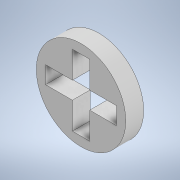
# Autodesk Inventor part: rod_7
Saved by Autodesk Inventor 2022 (Build 260153000, 153)
## iProperties
Created: 2023-04-14
Part Number: rod_7
Material: 一般
Document SubType Name: Modeling
Designer: Johnny Jou
Density: 1 g/cm^3
Appearance: 預設
Author: Johnny Jou
Autodesk Inventor part; units mm, degrees
ref_plane "YZ Plane" through (0, 0, 0) normal (1, 0, 0) x (0, 1, 0)
ref_plane "XZ Plane" through (0, 0, 0) normal (0, 1, 0) x (-1, 0, 0)
ref_plane "XY Plane" through (0, 0, 0) normal (0, 0, 1) x (1, 0, 0)
sketch "草圖1" plane through (0, 0, 0) normal (0, 0, 1) x (1, 0, 0)
  circle A0 centre (0, 0) radius 7.5
  line L0 (5.95, -1.45) -> (-5.95, -1.45)
  line L1 (-5.95, -1.45) -> (-5.95, 1.45)
  line L2 (-5.95, 1.45) -> (5.95, 1.45)
  line L3 (5.95, 1.45) -> (5.95, -1.45)
  line L4 (5.95, -1.45) -> (-5.95, 1.45) construction
  line L5 (-5.95, -1.45) -> (5.95, 1.45) construction
  line L6 (1.45, -5.95) -> (-1.45, -5.95)
  line L7 (-1.45, -5.95) -> (-1.45, 5.95)
  line L8 (-1.45, 5.95) -> (1.45, 5.95)
  line L9 (1.45, 5.95) -> (1.45, -5.95)
  line L10 (1.45, -5.95) -> (-1.45, 5.95) construction
  line L11 (-1.45, -5.95) -> (1.45, 5.95) construction
  point P0 (-1.45, 1.45)
  point P1 (1.45, 1.45)
  point P2 (1.45, -1.45)
  point P3 (-1.45, -1.45)
  dimension "d0" = 15
  dimension "d1" = 11.9
  dimension "d2" = 2.9
  constraints: 24 end point, 4 midpoint, 4 parallel, 4 perpendicular, 2 horizontal, 1 centre point, 1 coincident
  measures "d0" diameter of A0
  measures "d1" distance of L1.end L2.end
  measures "d2" distance of L0.end L1.end
extrude "擠出1" add sketch "草圖1" along normal blind 3
